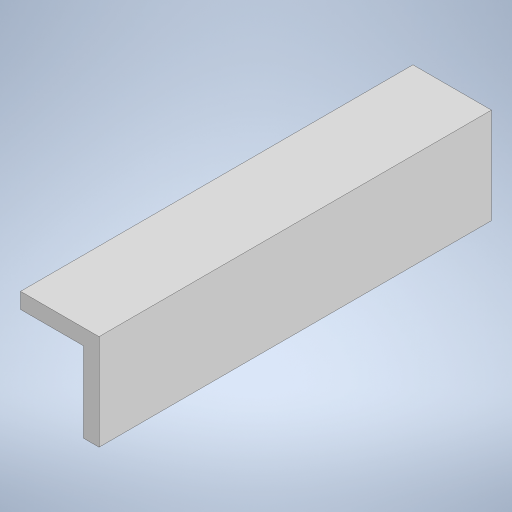
# Autodesk Inventor part: рельса крышечки
Saved by Autodesk Inventor 2023.1 (Build 271208000, 208)
## iProperties
Created: 2023-04-14
Part Number: рельса крышечки
Material: Типовые
Document SubType Name: Modeling
Designer: User
Density: 1 g/cm^3
Appearance: По умолчанию
Author: User
Autodesk Inventor part; units mm, degrees
ref_plane "YZ Plane" through (0, 0, 0) normal (1, 0, 0) x (0, 1, 0)
ref_plane "XZ Plane" through (0, 0, 0) normal (0, 1, 0) x (-1, 0, 0)
ref_plane "XY Plane" through (0, 0, 0) normal (0, 0, 1) x (1, 0, 0)
sketch "Эскиз1" plane through (0, 0, 0) normal (0, 0, 1) x (1, 0, 0)
  line L0 (0, 0) -> (1, 0)
  line L1 (1, 0) -> (1, 6.1)
  line L2 (1, 6.1) -> (0, 6.1)
  line L3 (0, 5.1) -> (0, 0)
  line L4 (1, 6.1) -> (-4, 6.1)
  line L5 (-4, 6.1) -> (-4, 5.1)
  line L6 (-4, 5.1) -> (0, 5.1)
  line L7 (1, 5.1) -> (1, 6.1)
  point P0 (0.5, 0)
  dimension "d0" = 6.1
  dimension "d1" = 5.1
  dimension "d2" = 4
  dimension "d3" = 1
  constraints: 16 end point, 4 parallel, 2 horizontal, 2 perpendicular, 1 midpoint
  measures "d0" distance between parallel lines of L2 L0
  measures "d1" distance from line of point (0.5, 0) L6
  measures "d2" distance between parallel lines of L3 L5
  measures "d3" distance between parallel lines of L1 L3
extrude "Выдавливание1" add sketch "Эскиз1" along normal blind 25
